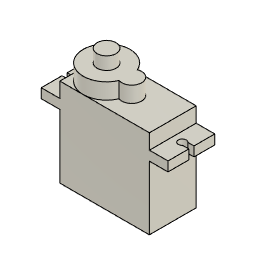
SG90 v1 (Autodesk Fusion 360 design; units mm, degrees)
Autodesk Fusion 360 part; units mm, degrees
note: some values were not read from the file. Set by a fixed rule: which sketch regions a step uses.
sketch "Sketch1" plane through (0, 0, 0) normal (0, 0, 1) x (1, 0, 0)
  line L0 (0, 0) -> (-22.6, 0)
  line L1 (-22.6, 0) -> (-22.6, 22.3)
  line L2 (-22.6, 22.3) -> (0, 22.3)
  line L3 (0, 22.3) -> (0, 0)
  line L4 (-22.6, 16.1) -> (-27.3, 16.1)
  line L5 (-27.3, 16.1) -> (-27.3, 18.5)
  line L6 (-27.3, 18.5) -> (-22.6, 18.5)
  line L7 (-11.3, 22.3) -> (-11.3, 0) construction
  line L8 (0, 16.1) -> (4.7, 16.1)
  line L9 (4.7, 16.1) -> (4.7, 18.5)
  line L10 (4.7, 18.5) -> (0, 18.5)
  dimension "d1" = 22.6
  dimension "d2" = 22.3
  dimension "d3" = 16.1
  dimension "d4" = 2.4
  dimension "d5" = 4.7
  constraint horizontal L0
  constraint vertical L1
  constraint horizontal L2
  constraint vertical L3
  constraint coincident L0.start L3.end
  constraint coincident L1 L4.start
  constraint perpendicular L1 L4
  constraint perpendicular L4 L5
  constraint coincident L1 L6.end
  constraint perpendicular L1 L6
  constraint midpoint L2 L7.start
  constraint midpoint L0 L7.end
  constraint symmetric L4.start L7 L8.start
  constraint symmetric L4.end L7 L8.end
  constraint symmetric L5.end L7 L9.end
  constraint symmetric L6.end L7 L10.end
  measures "d1" distance of L0.start L0.end
  measures "d2" distance of L0.start L2.end
  measures "d3" distance of L0.end L4
  measures "d4" distance of L4.end L5.end
  measures "d5" distance of L5.end L6.end
extrude "Extrude1" add sketch "Sketch1" along normal blind 11.8
sketch "Sketch2" plane through (0, 22.3, 0) normal (0, 1, 0) x (-1, 0, 0)
  line L0 (0, 0) -> (22.6, 0)
  line L1 (22.6, 0) -> (22.6, 11.8)
  line L2 (22.6, 11.8) -> (0, 11.8)
  line L3 (0, 11.8) -> (0, 0)
  circle A0 centre (16.7, 5.9) radius 5.9
  circle A1 centre (16.7, 5.9) radius 2.4
  line L4 (16.7, 5.9) -> (7.9, 5.9) construction
  circle A2 centre (10.3996, 5.8553) radius 2.5
  dimension "d8" = 4.8
  dimension "d13" = 8.8
  dimension "d14" = 5
  constraint tangent L2 A0
  constraint tangent L0 A0
  constraint tangent L1 A0
  constraint concentric A0 A1
  constraint coincident A0.centre A1.centre
  constraint horizontal L4
  constraint coincident L4.end A2
  measures "d8" diameter of A1
  measures "d13" distance of A0.centre L4.end
  measures "d14" diameter of A2
extrude "Extrude2" add sketch "Sketch2" along normal blind 4 contours A0 A2 | A0 A2 | A0 A2
extrude "Extrude3" add sketch "Sketch2" along normal blind 7.2 contours A1
sketch "Sketch3" plane through (0, 18.5, 0) normal (0, 1, 0) x (-1, 0, 0)
  line L0 (-4.7, 0) -> (0, 0)
  line L1 (0, 0) -> (0, 11.8)
  line L2 (0, 11.8) -> (-4.7, 11.8)
  line L3 (-4.7, 11.8) -> (-4.7, 0)
  line L4 (22.6, 0) -> (27.3, 0)
  line L5 (27.3, 0) -> (27.3, 11.8)
  line L6 (27.3, 11.8) -> (22.6, 11.8)
  line L7 (22.6, 11.8) -> (22.6, 0)
  line L8 (0, 11.8) -> (16.7, 11.8)
  line L9 (16.7, 11.8) -> (22.6, 11.8)
  line L10 (0, 11.8) -> (22.6, 11.8) construction
  line L11 (11.3, 11.8) -> (11.3, 0) construction
  line L12 (-4.7, 5.9) -> (-2.4, 5.9) construction
  circle A0 centre (-2.4, 5.9) radius 1
  circle A1 centre (25, 5.9) radius 1
  line L13 (-4.7, 5.25) -> (-2.4, 5.25)
  line L14 (-4.7, 6.55) -> (-2.4, 6.55)
  line L15 (27.3, 6.55) -> (25, 6.55)
  line L16 (27.3, 5.25) -> (25, 5.25)
  dimension "d15" = 2.3
  dimension "d16" = 2
  dimension "d17" = 0.65
  dimension "d18" = -0.65
  constraint coincident L1.end L2.start
  constraint coincident L6.end L7.start
  constraint midpoint L10 L11.start
  constraint perpendicular L8 L11
  constraint midpoint L3 L12.start
  constraint perpendicular L1 L12
  constraint coincident L12.end A0.centre
  constraint symmetric L11 A0 A1
  constraint symmetric L11 L13.start L16.start
  constraint symmetric L11 L13.end L16.end
  constraint symmetric L11 L14.start L15.start
  constraint symmetric L11 L14.end L15.end
  measures "d15" distance of L12.start L12.end
  measures "d16" diameter of A0
extrude "Extrude4" cut sketch "Sketch3" against normal blind 2.4 contours L3 A0 L13 L14 | A0 | L5 A1 L15 L16 | A1
move_body "Move1" bodies 1 to x (1, 0, 0) y (0, 0, 1) z (0, -1, 0) at (0, 0, 0)
move_body "Move2" bodies 1 to x (1, 0, 0) y (0, 1, 0) z (0, 0, 1) at (11.3, 5.9, 0)
equation "d5 = ( ( 31.8 - 22.4 ) / 2 ) * 1 mm"
